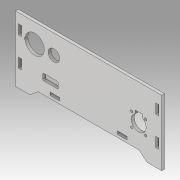
# Autodesk Inventor part: front_instrumentboard
Saved by Autodesk Inventor 2019.3 (Build 233278000, 278)
## iProperties
Created: 2019-05-28
Part Number: front_instrumentboard
Material: Generic
Document SubType Name: Modeling
Designer: Dave
Density: 1 g/cm^3
Appearance: Default
Author: Dave
Autodesk Inventor part; units mm, degrees
ref_plane "YZ Plane" through (0, 0, 0) normal (1, 0, 0) x (0, 1, 0)
ref_plane "XZ Plane" through (0, 0, 0) normal (0, 1, 0) x (-1, 0, 0)
ref_plane "XY Plane" through (0, 0, 0) normal (0, 0, 1) x (1, 0, 0)
sketch "Sketch1" plane through (0, 0, 0) normal (0, 0, 1) x (1, 0, 0)
  line L0 (0, 0) -> (152, 0)
  line L1 (152, 0) -> (152, 68)
  line L2 (152, 68) -> (0, 68)
  line L3 (0, 68) -> (0, 0)
  line L4 (36, 13) -> (46, 13)
  line L5 (46, 13) -> (46, 10)
  line L6 (46, 10) -> (36, 10)
  line L7 (36, 10) -> (36, 13)
  line L8 (106, 13) -> (116, 13)
  line L9 (116, 13) -> (116, 10)
  line L10 (116, 10) -> (106, 10)
  line L11 (106, 10) -> (106, 13)
  line L12 (3, 28) -> (6.1, 28)
  line L13 (6.1, 28) -> (6.1, 18)
  line L14 (6.1, 18) -> (3, 18)
  line L15 (3, 18) -> (3, 28)
  line L16 (3, 58) -> (6.1, 58)
  line L17 (6.1, 58) -> (6.1, 48)
  line L18 (6.1, 48) -> (3, 48)
  line L19 (3, 48) -> (3, 58)
  line L20 (145.9, 58) -> (149, 58)
  line L21 (149, 58) -> (149, 48)
  line L22 (149, 48) -> (145.9, 48)
  line L23 (145.9, 48) -> (145.9, 58)
  line L24 (145.9, 28) -> (149, 28)
  line L25 (149, 28) -> (149, 18)
  line L26 (149, 18) -> (145.9, 18)
  line L27 (145.9, 18) -> (145.9, 28)
  line L28 (23.5, 7) -> (128.5, 7)
  line L29 (128.5, 7) -> (137, 0)
  line L30 (23.5, 7) -> (15, 0)
  dimension "d0" = 3
  dimension "d1" = 10
  dimension "d2" = 60
  dimension "d3" = 10
  dimension "d4" = 152
  dimension "d5" = 36
  dimension "d6" = 36
  dimension "d7" = 3.1
  dimension "d8" = 10
  dimension "d9" = 20
  dimension "d10" = 5
  dimension "d11" = 10
  dimension "d12" = 3
  dimension "d13" = 3
  dimension "d14" = 3
  dimension "d15" = 15
  dimension "d16" = 15
  dimension "d17" = 105
  constraints: 62 end point, 14 parallel, 8 horizontal, 8 point on line, 7 perpendicular, 6 equal length, 2 collinear
  measures "d0" distance of L6.end L4.start
  measures "d1" distance of L4.start L4.end
  measures "d2" distance between parallel lines of L11 L5
  measures "d3" distance between parallel lines of L0 L6
  measures "d4" distance between parallel lines of L1 L3
  measures "d5" distance between parallel lines of L1 L9
  measures "d6" distance between parallel lines of L3 L7
  measures "d7" distance of L16.start L16.end
  measures "d8" distance of L16.end L17.end
  measures "d9" distance between parallel lines of L12 L18
  measures "d10" distance between parallel lines of L4 L14
  measures "d11" distance between parallel lines of L2 L16
  measures "d12" distance between parallel lines of L1 L21
  measures "d13" distance between parallel lines of L3 L19
  measures "d14" distance between parallel lines of L28 L6
  measures "d15" distance from line of L3 L30.end
  measures "d16" distance from line of L1 L29.end
  measures "d17" distance of L28.start L28.end
extrude "Extrusion1" add sketch "Sketch1" along normal blind 3 contours L3 L2 L1 L0 L29 L28 L30
sketch "Sketch2" plane through (0, 0, 3) normal (0, 0, 1) x (1, 0, 0)
  line L0 (29.5, 26.41) -> (43.5, 26.41)
  line L1 (44.5, 25.41) -> (44.5, 20.83)
  line L2 (43.5, 19.83) -> (29.5, 19.83)
  line L3 (28.5, 20.83) -> (28.5, 25.41)
  line L4 (145.9, 18) -> (145.9, 28) projected
  line L5 (106, 13) -> (116, 13) projected
  line L6 (6.1, 28) -> (6.1, 18) projected
  line L7 (3, 28) -> (6.1, 28) projected
  line L8 (6.1, 18) -> (3, 18) projected
  arc A0 (29.5, 26.41) -> (28.5, 25.41) centre (29.5, 25.41) ccw
  arc A1 (28.5, 20.83) -> (29.5, 19.83) centre (29.5, 20.83) ccw
  arc A2 (43.5, 19.83) -> (44.5, 20.83) centre (43.5, 20.83) ccw
  arc A3 (44.5, 25.41) -> (43.5, 26.41) centre (43.5, 25.41) ccw
  line L9 (46, 10) -> (36, 10) projected
  arc A4 (124.65, 37.6647) -> (131.65, 37.6647) centre (128.15, 30.75) ccw
  line L10 (124.65, 41) -> (131.65, 41)
  line L11 (131.65, 41) -> (131.65, 37.6647)
  line L12 (124.65, 37.6647) -> (124.65, 41)
  circle A5 centre (120.9, 38) radius 1.25
  circle A6 centre (135.4, 38) radius 1.25
  circle A7 centre (135.4, 23.5) radius 1.25
  circle A8 centre (120.9, 23.5) radius 1.25
  circle A9 centre (128.15, 30.75) radius 10.253 construction
  point P0 (0, 0)
  point P1 (28.5, 26.41)
  point P2 (44.5, 19.83)
  point P3 (44.5, 26.41)
  point P4 (28.5, 19.83)
  point P5 (128.15, 41)
  dimension "d21" = 16
  dimension "d26" = 22.4
  dimension "d29" = 1
  dimension "d30" = 6.58
  dimension "d31" = 9.83
  dimension "d32" = 15.5
  dimension "d33" = 7
  dimension "d34" = 18
  dimension "d35" = 2.5
  dimension "d36" = 17
  dimension "d37" = 17
  dimension "d38" = 10.253
  dimension "d39" = 10.253
  dimension "d40" = 10.253
  dimension "d41" = 17.75
  dimension "d42" = 10
  dimension "d43" = 17.75
  constraints: 14 end point, 13 point on circle, 10 centre point, 8 point on line, 8 tangent, 6 equal radius, 3 parallel, 3 vertical alignment, 2 horizontal, 2 horizontal alignment, 2 perpendicular, 1 coincident, 1 midpoint
  measures "d21" distance of point (28.5, 26.41) point (44.5, 26.41)
  measures "d26" distance between parallel lines of L6 L3
  measures "d29" radius of A0
  measures "d30" distance between parallel lines of L0 L2
  measures "d31" distance between parallel lines of L9 L2
  measures "d32" diameter of A4
  measures "d33" distance of L10.start L10.end
  measures "d35" diameter of A5
  measures "d38" distance of A4.centre A5.centre
  measures "d39" distance of A7.centre A4.centre
  measures "d40" distance of A4.centre A6.centre
  measures "d41" distance from line of L4 A4.centre
  measures "d42" distance edge to line of A4 L4
  measures "d43" distance from line of L5 A4.centre
extrude "Extrusion2" cut sketch "Sketch2" against normal blind 10
sketch "Sketch3" plane through (0, 0, 3) normal (0, 0, 1) x (1, 0, 0)
  circle A0 centre (40, 48) radius 6
  arc A1 (10.0501, 47) -> (10.0501, 49) centre (20, 48) ccw
  line L0 (0, 68) -> (0, 0) projected
  line L1 (9.2, 49) -> (10.0501, 49)
  line L2 (10.0501, 47) -> (9.2, 47)
  line L3 (9.2, 47) -> (9.2, 49)
  line L4 (152, 68) -> (0, 68) projected
  point P0 (10.0501, 48)
  point P1 (9.2, 48)
  dimension "d44" = 12
  dimension "d45" = 20
  dimension "d46" = 20
  dimension "d47" = 20
  dimension "d48" = 2
  dimension "d49" = 10.8
  dimension "d50" = 20
  dimension "d51" = 10.0501
  constraints: 6 end point, 3 horizontal alignment, 2 centre point, 2 parallel, 2 point on circle, 1 horizontal, 1 midpoint
  measures "d44" diameter of A0
  measures "d45" diameter of A1
  measures "d46" distance of A0.centre A1.centre
  measures "d47" distance from line of L0 A1.centre
  measures "d48" distance between parallel lines of L2 L1
  measures "d49" distance from line of A1.centre L3
  measures "d50" distance from line of L4 A1.centre
  measures "d51" distance from line of point (10.05, 48) L0
extrude "Extrusion3" cut sketch "Sketch3" against normal blind 10
body "Solid1"
